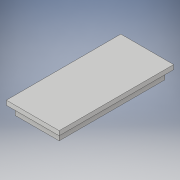
# Autodesk Inventor part: Caja_Superior
Saved by Autodesk Inventor 2019 (Build 230136000, 136)
## iProperties
Created: 2020-07-21
Part Number: Caja_Superior
Material: Generic
Document SubType Name: Modeling
Designer: Sergio
Density: 1 g/cm^3
Appearance: Default
Author: Sergio
Autodesk Inventor part; units mm, degrees
ref_plane "YZ Plane" through (0, 0, 0) normal (1, 0, 0) x (0, 1, 0)
ref_plane "XZ Plane" through (0, 0, 0) normal (0, 1, 0) x (-1, 0, 0)
ref_plane "XY Plane" through (0, 0, 0) normal (0, 0, 1) x (1, 0, 0)
sketch "Sketch1" plane through (0, 0, 0) normal (0, 1, 0) x (-1, 0, 0)
  line L0 (-25, -60) -> (25, -60)
  line L1 (25, -60) -> (25, 60)
  line L2 (25, 60) -> (-25, 60)
  line L3 (-25, 60) -> (-25, -60)
  line L4 (-25, -60) -> (25, 60) construction
  line L5 (25, -60) -> (-25, 60) construction
  point P0 (0, 0)
  dimension "d0" = 50
  dimension "d1" = 120
  constraints: 12 end point, 2 midpoint, 2 parallel, 1 horizontal, 1 perpendicular
  measures "d0" distance of L2.end L1.end
  measures "d1" distance of L1.end L0.end
extrude "Extrusion1" add sketch "Sketch1" against normal blind 10
sketch "Sketch2" plane through (0, 0, 0) normal (0, 1, 0) x (1, 0, 0)
  line L0 (30, 65) -> (-30, 65)
  line L1 (-30, 65) -> (-30, -65)
  line L2 (-30, -65) -> (30, -65)
  line L3 (30, -65) -> (30, 65)
  line L4 (30, 65) -> (-30, -65) construction
  line L5 (-30, 65) -> (30, -65) construction
  point P0 (0, 0)
  dimension "d4" = 60
  dimension "d5" = 130
  constraints: 12 end point, 2 midpoint, 2 parallel, 1 horizontal, 1 perpendicular
  measures "d4" distance of L2.end L1.end
  measures "d5" distance of L1.end L0.end
extrude "Extrusion2" add sketch "Sketch2" along normal blind 5
body "Solid1"
